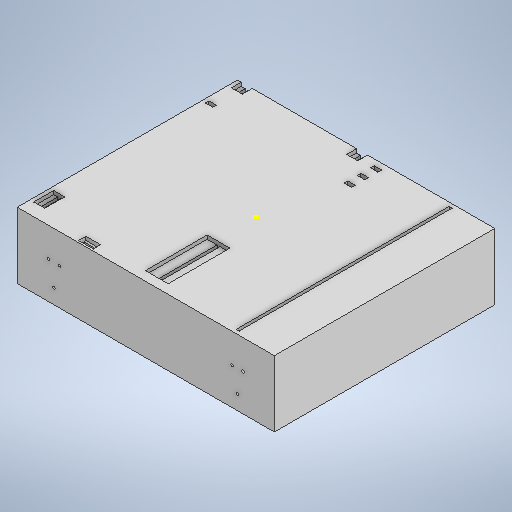
# Autodesk Inventor part: Venstre
Saved by Autodesk Inventor 2025.2 (Build 292293000, 293)
## iProperties
Created: 2025-05-06
Part Number: Venstre
Material: Generic
Document SubType Name: Modeling
Designer: lauri
Density: 1 g/cm^3
Appearance: Default
Author: lauri
Autodesk Inventor part; units mm, degrees
ref_plane "YZ Plane" through (0, 0, 0) normal (1, 0, 0) x (0, 1, 0)
ref_plane "XZ Plane" through (0, 0, 0) normal (0, 1, 0) x (-1, 0, 0)
ref_plane "XY Plane" through (0, 0, 0) normal (0, 0, 1) x (1, 0, 0)
sketch "Sketch2" plane through (0, 0, 0) normal (0, 1, 0) x (-1, 0, 0)
  line L0 (-175, 150) -> (175, 150)
  line L1 (175, 150) -> (175, -150)
  line L2 (175, -150) -> (-175, -150)
  line L3 (-175, -150) -> (-175, 150)
  line L4 (-175, 150) -> (175, -150) construction
  line L5 (175, 150) -> (-175, -150) construction
  point P0 (0, 0)
  dimension "d6" = 350
  dimension "d7" = 300
  constraints: 12 end point, 2 midpoint, 2 parallel, 1 horizontal, 1 perpendicular
  measures "d6" distance of L1.end L2.end
  measures "d7" distance of L0.end L1.end
extrude "Extrusion1" add sketch "Sketch2" along normal blind 10
sketch "Sketch4" plane through (0, 10, 0) normal (0, 1, 0) x (1, 0, 0)
  line L0 (-175, -150) -> (175, -150) projected
  line L1 (-170, -132.5) -> (-155, -132.5)
  line L2 (-155, -132.5) -> (-155, -105.5)
  line L3 (-155, -105.5) -> (-170, -105.5)
  line L4 (-170, -105.5) -> (-170, -132.5)
  point P0 (0, 0)
  point P1 (-170, -142.5)
  point P2 (-13, -145)
  point P3 (-170, -142.5)
  dimension "d122" = 15
  dimension "d123" = 27
  constraints: 8 end point, 2 parallel, 1 horizontal, 1 perpendicular
  measures "d122" distance of L3.end L2.end
  measures "d123" distance of L2.end L1.end
sketch "Sketch5" plane through (0, 10, 0) normal (0, 1, 0) x (1, 0, 0)
  line L0 (-155, -117.5) -> (-155, -142.5) projected
  line L1 (-175, -150) -> (175, -150) projected
  line L2 (-13, -137.5) -> (18, -137.5)
  line L3 (18, -137.5) -> (18, -53.5)
  line L4 (18, -53.5) -> (-13, -53.5)
  line L5 (-13, -137.5) -> (-13, -53.5)
  point P0 (0, 0)
  dimension "d24" = 31
  dimension "d25" = 84
  constraints: 8 end point, 1 coincident, 1 horizontal, 1 parallel, 1 perpendicular, 1 vertical
  measures "d24" distance of L4.end L3.end
  measures "d25" distance of L3.end L2.end
extrude "Extrusion3" cut sketch "Sketch5" against normal blind 5
sketch "Sketch7" plane through (0, 10, 0) normal (0, 1, 0) x (1, 0, 0)
  line L0 (-13, -53.5) -> (18, -53.5) projected
  line L1 (175, 150) -> (-175, 150) projected
  line L2 (-170, 150) -> (-155, 150)
  line L3 (-155, 150) -> (-155, 136.5)
  line L4 (-155, 136.5) -> (-170, 136.5)
  line L5 (-170, 136.5) -> (-170, 150)
  line L6 (-13, 136.5) -> (2, 136.5)
  line L7 (2, 136.5) -> (2, 150)
  line L8 (2, 150) -> (-13, 150)
  line L9 (-13, 150) -> (-13, 136.5)
  point P0 (0, 0)
  point P1 (-13, -63.5)
  point P2 (-170, -117.5)
  point P3 (-155, 150)
  point P4 (-170, 150)
  dimension "d34" = 15
  dimension "d35" = 13.5
  dimension "d39" = 15
  dimension "d53" = 13.5
  constraints: 16 end point, 4 parallel, 2 horizontal, 2 perpendicular, 2 point on line, 1 other
  measures "d34" distance of L3.end L4.end
  measures "d35" distance of L2.end L3.end
  measures "d39" distance of L8.end L7.end
  measures "d53" distance of L6.end L7.end
extrude "Extrusion6" cut sketch "Sketch7" against normal blind 5
sketch "Sketch8" plane through (0, 5, 0) normal (0, 1, 0) x (1, 0, 0)
  line L0 (2, 150) -> (2, 136.5) projected
  line L1 (-13, 136.5) -> (-13, 150) projected
  line L2 (-3.5, 136.5) -> (-7.5, 136.5)
  line L3 (-7.5, 136.5) -> (-7.5, 150)
  line L4 (-7.5, 150) -> (-3.5, 150)
  line L5 (-3.5, 150) -> (-3.5, 136.5)
  line L6 (-3.5, 136.5) -> (-7.5, 150) construction
  line L7 (-7.5, 136.5) -> (-3.5, 150) construction
  line L8 (-170, 136.5) -> (-170, 150) projected
  line L9 (-170, 143.25) -> (-155, 143.25)
  line L10 (-155, 150) -> (-155, 136.5) projected
  line L11 (-164.5, 136.5) -> (-160.5, 136.5)
  line L12 (-160.5, 136.5) -> (-160.5, 150)
  line L13 (-160.5, 150) -> (-164.5, 150)
  line L14 (-164.5, 150) -> (-164.5, 136.5)
  line L15 (-164.5, 136.5) -> (-160.5, 150) construction
  line L16 (-160.5, 136.5) -> (-164.5, 150) construction
  point P0 (0, 0)
  point P1 (-5.5, 143.25)
  point P2 (-162.5, 143.25)
  dimension "d42" = 4
  dimension "d43" = 13.5
  dimension "d44" = 4
  dimension "d45" = 13.5
  constraints: 26 end point, 7 midpoint, 4 parallel, 2 horizontal, 2 perpendicular
  measures "d42" distance of L3.end L4.end
  measures "d43" distance of L2.end L3.end
  measures "d44" distance of L13.end L12.end
  measures "d45" distance of L12.end L11.end
extrude "Extrusion7" cut sketch "Sketch8" against normal through all
sketch "Sketch9" plane through (0, 10, 0) normal (0, 1, 0) x (1, 0, 0)
  point P0 (0, 0)
sketch "Sketch12" plane through (0, 10, 0) normal (0, 1, 0) x (1, 0, 0)
  line L0 (-175, -150) -> (175, -150) projected
  line L1 (175, -150) -> (175, -145)
  line L2 (175, -150) -> (175, 150) projected
  line L3 (175, -145) -> (120, -145)
  line L4 (118, 145) -> (122, 145)
  line L5 (122, 145) -> (122, -145)
  line L6 (122, -145) -> (118, -145)
  line L7 (118, -145) -> (118, 145)
  line L8 (118, 145) -> (122, -145) construction
  line L9 (122, 145) -> (118, -145) construction
  point P0 (0, 0)
  point P1 (120, 0)
  dimension "d57" = 5
  dimension "d58" = 55
  dimension "d59" = 4
  constraints: 16 end point, 2 midpoint, 2 parallel, 2 perpendicular, 2 point on line, 1 horizontal
  measures "d57" distance of L0.end L1.end
  measures "d58" distance of L1.end L3.end
  measures "d59" distance of L5.end L6.end
extrude "Extrusion11" cut sketch "Sketch12" against normal blind 10
sketch "Sketch13" plane through (0, 0, 0) normal (0, -1, 0) x (1, 0, 0)
  line L0 (-175, 150) -> (175, 150) projected
  line L1 (175, -150) -> (170, -150)
  line L2 (170, -150) -> (170, 150)
  line L3 (170, 150) -> (175, 150)
  line L4 (175, 150) -> (175, -150)
  line L5 (-175, -150) -> (-175, 150) projected
  line L6 (175, 150) -> (-175, 150)
  line L7 (-175, 150) -> (-175, 145)
  line L8 (-175, 145) -> (175, 145)
  line L9 (175, 145) -> (175, 150)
  line L10 (-175, 150) -> (-170, 150)
  line L11 (-170, 150) -> (-170, -150)
  line L12 (-170, -150) -> (-175, -150)
  line L13 (-175, -150) -> (-175, 150)
  point P0 (0, 0)
  point P1 (175, 150)
  point P2 (-170, 145)
  point P3 (170, 145)
  dimension "d62" = 5
  dimension "d63" = 5
  dimension "d64" = 5
  constraints: 24 end point, 6 parallel, 3 horizontal, 3 perpendicular, 3 point on line
  measures "d62" distance of L2.end L3.end
  measures "d63" distance of L7.end L6.end
  measures "d64" distance of L11.end L12.end
extrude "Extrusion12" add sketch "Sketch13" along normal blind 80
sketch "Sketch14" plane through (0, 10, 0) normal (0, 1, 0) x (1, 0, 0)
  line L0 (2, 150) -> (2, 136.5) projected
  line L1 (2, 150) -> (19, 150)
  line L2 (170, 150) -> (-3.5, 150) projected
  line L3 (19, 150) -> (19, 141.9)
  line L4 (19, 141.9) -> (29, 141.9)
  line L5 (29, 141.9) -> (29, 136.9)
  line L6 (29, 136.9) -> (19, 136.9)
  line L7 (19, 136.9) -> (19, 141.9)
  line L8 (19, 123.9) -> (29, 123.9)
  line L9 (29, 123.9) -> (29, 118.9)
  line L10 (29, 118.9) -> (19, 118.9)
  line L11 (19, 118.9) -> (19, 123.9)
  line L12 (19, 121.4) -> (19, 105.9)
  line L13 (19, 105.9) -> (29, 105.9)
  line L14 (29, 105.9) -> (29, 100.9)
  line L15 (29, 100.9) -> (19, 100.9)
  line L16 (19, 100.9) -> (19, 105.9)
  line L17 (-170, 150) -> (-170, -145) projected
  line L18 (-170, 105.9) -> (-160, 105.9)
  line L19 (-160, 105.9) -> (-160, 100.9)
  line L20 (-160, 100.9) -> (-170, 100.9)
  line L21 (-170, 100.9) -> (-170, 105.9)
  point P0 (0, 0)
  dimension "d67" = 17
  dimension "d68" = 8.1
  dimension "d70" = 5
  dimension "d72" = 5
  dimension "d73" = 15.5
  dimension "d74" = 5
  dimension "d75" = 10
  constraints: 38 end point, 8 parallel, 5 perpendicular, 4 horizontal, 3 point on line, 1 midpoint
  measures "d67" distance of L0.start L1.end
  measures "d68" distance of L1.end L3.end
  measures "d70" distance of L4.end L5.end
  measures "d72" distance of L8.end L9.end
  measures "d73" distance of L12.start L12.end
  measures "d74" distance of L13.end L14.end
  measures "d75" distance of L19.end L20.end
extrude "Extrusion13" cut sketch "Sketch14" against normal blind 5
sketch "Sketch15" plane through (0, 10, 0) normal (0, 1, 0) x (1, 0, 0)
  line L0 (29, 123.9) -> (29, 118.9) projected
  line L1 (29, 121.4) -> (26.483, 121.4)
  line L2 (29, 105.9) -> (29, 100.9) projected
  line L3 (29, 103.4) -> (26.483, 103.4)
  line L4 (29, 141.9) -> (29, 136.9) projected
  line L5 (29, 139.4) -> (26.483, 139.4)
  line L6 (-170, 150) -> (-170, -145) projected
  line L7 (-170, 103.4) -> (-170, 105.917)
  line L8 (-170, 103.4) -> (-167.483, 103.4)
  point P0 (0, 0)
  dimension "d78" = 2.517
  dimension "d79" = 2.517
  dimension "d80" = 2.517
  dimension "d81" = 2.517
  dimension "d82" = 2.517
  constraints: 10 end point, 3 horizontal, 3 midpoint, 2 point on line, 1 perpendicular
  measures "d78" distance of L1.start L1.end
  measures "d79" distance of L3.start L3.end
  measures "d80" distance of L5.start L5.end
  measures "d81" distance of L7.start L7.end
  measures "d82" distance of L7.start L8.end
hole "Hole1" at (26.483, 10, -139.4) at (26.483, 10, -121.4) at (26.483, 10, -103.4) at (-167.483, 10, -103.4) direction (0, -1, 0) diameter 3.5 end through all
sketch "Sketch16" plane through (0, 0, 0) normal (0, -1, 0) x (1, 0, 0)
  line L0 (170, -150) -> (170, 145) projected
  line L1 (170, -150) -> (140, -150)
  line L2 (175, -150) -> (2, -150) projected
  line L3 (140, -150) -> (110, -150)
  line L4 (110, -150) -> (110, -145)
  line L5 (110, -145) -> (140, -145)
  line L6 (140, -145) -> (140, -150)
  line L7 (-170, 145) -> (-170, -150) projected
  line L8 (-170, -150) -> (-140, -150)
  line L9 (-7.5, -150) -> (-160.5, -150) projected
  line L10 (-140, -150) -> (-110, -150)
  line L11 (-110, -150) -> (-110, -145)
  line L12 (-110, -145) -> (-140, -145)
  line L13 (-140, -145) -> (-140, -150)
  point P0 (0, 0)
  dimension "d90" = 30
  dimension "d91" = 30
  dimension "d92" = 5
  dimension "d93" = 30
  dimension "d94" = 30
  constraints: 20 end point, 4 parallel, 2 horizontal, 2 perpendicular, 2 point on line
  measures "d90" distance of L0.start L1.end
  measures "d91" distance of L4.end L5.end
  measures "d92" distance of L3.end L4.end
  measures "d93" distance of L7.end L8.end
  measures "d94" distance of L12.end L11.end
extrude "Extrusion14" add sketch "Sketch16" along normal blind 20
sketch "Sketch17" plane through (-13, 10, -150) normal (0, 0, -1) x (-1, 0, 0)
  line L0 (-153, -10) -> (-153, -30) projected
  line L1 (-153, -20) -> (-123, -20)
  line L2 (-123, -10) -> (-123, -30) projected
  line L3 (97, -10) -> (97, -30) projected
  line L4 (97, -20) -> (127, -20)
  line L5 (127, -10) -> (127, -30) projected
  point P0 (-13, -10)
  point P1 (-138, -20)
  point P2 (-145.5, -20)
  point P3 (-130.5, -20)
  point P4 (112, -20)
  point P5 (104.5, -20)
  point P6 (119.5, -20)
  constraints: 6 midpoint, 4 end point, 4 point on line
hole "Hole2" at (-132.5, -10, -150) at (-125, -10, -150) at (-117.5, -10, -150) at (117.5, -10, -150) at (125, -10, -150) at (132.5, -10, -150) direction (0, 0, 1) diameter 3.5 depth 5
sketch "Sketch18" plane through (-175, 10, 150) normal (0, 0, 1) x (1, 0, 0)
  line L0 (350, -90) -> (350, 0) projected
  line L1 (350, 0) -> (300, 0)
  line L2 (0, 0) -> (350, 0) projected
  line L3 (300, 0) -> (300, -70)
  line L4 (0, 0) -> (50, 0)
  line L5 (50, 0) -> (50, -70)
  point P0 (175, -10)
  point P1 (292.5, -40)
  point P2 (307.5, -40)
  point P3 (57.5, -40)
  point P4 (42.5, -40)
  dimension "d104" = 50
  dimension "d105" = 70
  dimension "d106" = 50
  dimension "d107" = 70
  constraints: 8 end point, 2 coincident, 2 perpendicular, 2 point on line
  measures "d104" distance of L0.end L1.end
  measures "d105" distance of L1.end L3.end
  measures "d106" distance of L2.start L4.end
  measures "d107" distance of L4.end L5.end
hole "Hole4" at (-132.5, -30, 150) at (-117.5, -30, 150) at (-125, -60, 150) at (132.5, -30, 150) at (117.5, -30, 150) at (125, -60, 150) direction (0, 0, -1) diameter 3.5 depth 5
extrude "Extrusion15" cut sketch "Sketch4" against normal blind 5
sketch "Sketch19" plane through (0, 10, 0) normal (0, 1, 0) x (1, 0, 0)
  line L0 (-170, -132.5) -> (-170, -105.5) projected
  line L1 (-170, -119) -> (-155, -119)
  line L2 (-155, -105.5) -> (-155, -132.5) projected
  line L3 (-170, -105.5) -> (-155, -105.5) projected
  line L4 (-164.5, -132.5) -> (-160.5, -132.5)
  line L5 (-160.5, -132.5) -> (-160.5, -105.5)
  line L6 (-160.5, -105.5) -> (-164.5, -105.5)
  line L7 (-164.5, -105.5) -> (-164.5, -132.5)
  line L8 (-164.5, -132.5) -> (-160.5, -105.5) construction
  line L9 (-160.5, -132.5) -> (-164.5, -105.5) construction
  point P0 (0, 0)
  point P1 (-162.5, -119)
  dimension "d126" = 4
  constraints: 14 end point, 5 midpoint, 2 parallel, 1 horizontal, 1 perpendicular, 1 point on line
  measures "d126" distance of L6.end L5.end
extrude "Extrusion16" cut sketch "Sketch19" against normal blind 10 contours L7 L3 L5 L1 | L1 L5 L4 L7
sketch "Sketch20" plane through (0, 10, 0) normal (0, 1, 0) x (1, 0, 0)
  line L0 (-13, -137.5) -> (-13, -53.5) projected
  line L1 (-13, -53.5) -> (18, -53.5) projected
  line L2 (4.5, -137.5) -> (0.5, -137.5)
  line L3 (0.5, -137.5) -> (0.5, -53.5)
  line L4 (0.5, -53.5) -> (4.5, -53.5)
  line L5 (4.5, -53.5) -> (4.5, -137.5)
  line L6 (4.5, -137.5) -> (0.5, -53.5) construction
  line L7 (0.5, -137.5) -> (4.5, -53.5) construction
  point P0 (0, 0)
  point P1 (2.5, -95.5)
  dimension "d129" = 4
  constraints: 12 end point, 2 midpoint, 2 parallel, 1 horizontal, 1 perpendicular, 1 point on line
  measures "d129" distance of L3.end L4.end
extrude "Extrusion17" cut sketch "Sketch20" against normal blind 10
sketch "Sketch21" plane through (0, 10, 0) normal (0, 1, 0) x (1, 0, 0)
  line L0 (18, -137.5) -> (-13, -137.5) projected
  line L1 (-13, -137.5) -> (-155, -137.5)
  line L2 (-84, -137.5) -> (-84, -142.5)
  line L3 (-74, -147.5) -> (-94, -147.5)
  line L4 (-94, -147.5) -> (-94, -137.5)
  line L5 (-94, -137.5) -> (-74, -137.5)
  line L6 (-74, -137.5) -> (-74, -147.5)
  line L7 (-74, -147.5) -> (-94, -137.5) construction
  line L8 (-94, -147.5) -> (-74, -137.5) construction
  point P0 (0, 0)
  dimension "d132" = 5
  dimension "d133" = 20
  constraints: 16 end point, 3 midpoint, 2 horizontal, 2 parallel, 1 perpendicular, 1 point on line, 1 vertical
  measures "d132" distance of L2.start L2.end
  measures "d133" distance of L4.end L5.end
extrude "Extrusion18" cut sketch "Sketch21" against normal blind 5
sketch "Sketch22" plane through (0, 10, 0) normal (0, 1, 0) x (1, 0, 0)
  line L0 (-94, -147.5) -> (-94, -137.5) projected
  line L1 (-94, -142.5) -> (-74, -142.5)
  line L2 (-74, -137.5) -> (-74, -147.5) projected
  line L3 (-74, -144.5) -> (-94, -144.5)
  line L4 (-94, -144.5) -> (-94, -140.5)
  line L5 (-94, -140.5) -> (-74, -140.5)
  line L6 (-74, -140.5) -> (-74, -144.5)
  line L7 (-74, -144.5) -> (-94, -140.5) construction
  line L8 (-94, -144.5) -> (-74, -140.5) construction
  point P0 (0, 0)
  point P1 (-84, -142.5)
  dimension "d136" = 4
  constraints: 14 end point, 5 midpoint, 2 parallel, 1 horizontal, 1 perpendicular, 1 point on line
  measures "d136" distance of L3.end L4.end
extrude "Extrusion19" cut sketch "Sketch22" against normal blind 10
body "Solid1"
